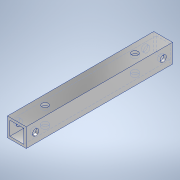
# Autodesk Inventor part: 上下直動9x9_3
Saved by Autodesk Inventor 2020.3 (Build 243373000, 373)
## iProperties
Created: 2020-07-05
Part Number: 上下直動9x9_3
Material: アルミニウム 6061
Document SubType Name: Modeling
Designer: totot
Density: 2.7 g/cm^3
Appearance: アルミニウム - フラット
Mass: 4.87118 g
Surface Area: 31.7226 cm^2
Volume: 1.80414 cm^3
Author: totot
Autodesk Inventor part; units mm, degrees
ref_plane "YZ Plane" through (0, 0, 0) normal (1, 0, 0) x (0, 1, 0)
ref_plane "XZ Plane" through (0, 0, 0) normal (0, 1, 0) x (-1, 0, 0)
ref_plane "XY Plane" through (0, 0, 0) normal (0, 0, 1) x (1, 0, 0)
sketch "スケッチ1" plane through (0, 0, 0) normal (0, 0, 1) x (1, 0, 0)
  line L0 (0, 0) -> (9, 0)
  line L1 (9, 0) -> (9, -9)
  line L2 (9, -9) -> (0, -9)
  line L3 (0, -9) -> (0, 0)
  line L4 (1.2, -1.2) -> (7.8, -1.2)
  line L5 (7.8, -1.2) -> (7.8, -7.8)
  line L6 (7.8, -7.8) -> (1.2, -7.8)
  line L7 (1.2, -7.8) -> (1.2, -1.2)
  dimension "d0" = 9
  dimension "d1" = 9
  dimension "d2" = 6.6
  dimension "d3" = 6.6
  dimension "d4" = 1.2
  dimension "d5" = 1.2
  constraints: 16 end point, 4 parallel, 2 horizontal, 2 perpendicular
  measures "d0" distance of L1.end L2.end
  measures "d1" distance of L0.end L1.end
  measures "d2" distance of L5.end L6.end
  measures "d3" distance of L4.end L5.end
  measures "d4" distance between parallel lines of L3 L7
  measures "d5" distance between parallel lines of L4 L0
extrude "押し出し1" add sketch "スケッチ1" along normal blind 75
sketch "スケッチ2" plane through (9, -9, 0) normal (1, 0, 0) x (0, 0, -1)
  line L0 (0, 9) -> (-75, 9) projected
  line L1 (0, 0) -> (0, 9) projected
  line L2 (-75, 0) -> (-75, 9) projected
  point P0 (-70.5, 4.5)
  point P1 (-4.5, 4.5)
  dimension "d8" = 4.5
  dimension "d9" = 4.5
  dimension "d10" = 4.5
  dimension "d11" = 4.5
  measures "d8" distance from line of point (-70.5, 4.5) L0
  measures "d9" distance from line of point (-4.5, 4.5) L0
  measures "d10" distance from line of point (-4.5, 4.5) L1
  measures "d11" distance from line of L2 point (-70.5, 4.5)
hole "穴1" at (9, -4.5, 70.5) at (9, -4.5, 4.5) direction (-1, 0, 0) diameter 3 end through all
sketch "スケッチ3" plane through (0, 0, 0) normal (0, 1, 0) x (1, 0, 0)
  line L0 (0, 0) -> (0, -75) projected
  line L1 (9, 0) -> (0, 0) projected
  line L2 (9, -75) -> (0, -75) projected
  point P0 (4.5, -61.5)
  point P1 (4.5, -13.5)
  dimension "d19" = 4.5
  dimension "d20" = 4.5
  dimension "d21" = 13.5
  dimension "d22" = 13.5
  measures "d19" distance from line of point (4.5, -61.5) L0
  measures "d20" distance from line of point (4.5, -13.5) L0
  measures "d21" distance from line of point (4.5, -13.5) L1
  measures "d22" distance from line of point (4.5, -61.5) L2
hole "穴2" at (4.5, 0, 61.5) at (4.5, 0, 13.5) direction (0, -1, 0) diameter 3 end through all
equation "\"d10\" = d9"
equation "\"d22\" = d21"
